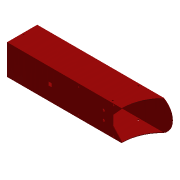
# Autodesk Inventor part: Case
Saved by Autodesk Inventor 2015 (Build 190159000, 159)
## iProperties
Created: 2015-01-07
Part Number: Case
Material: Všeobecné
Document SubType Name: Modeling
Designer: Michal
Density: 1 g/cm^3
Appearance: Červená
Author: Michal
Autodesk Inventor part; units mm, degrees
ref_plane "YZ Plane" through (0, 0, 0) normal (1, 0, 0) x (0, 1, 0)
ref_plane "XZ Plane" through (0, 0, 0) normal (0, 1, 0) x (-1, 0, 0)
ref_plane "XY Plane" through (0, 0, 0) normal (0, 0, 1) x (1, 0, 0)
sketch "Náčrt1" plane through (0, 0, 0) normal (1, 0, 0) x (0, 1, 0)
  line L0 (0, 0) -> (100, 0)
  line L1 (100, 0) -> (100, -100)
  line L2 (100, -100) -> (0, -100)
  line L3 (0, -100) -> (0, 0)
  line L4 (98, -2) -> (2, -2)
  line L5 (2, -2) -> (2, -98)
  line L6 (2, -98) -> (98, -98)
  line L7 (98, -98) -> (98, -2)
  dimension "d0" = 100
  dimension "d1" = 100
  dimension "d2" = 2
  constraints: 16 end point, 4 parallel, 2 perpendicular, 1 horizontal, 3 other
  measures "d0" distance of L1.end L2.end
  measures "d1" distance of L0.end L1.end
  measures "d2" distance between parallel lines of L0 L4
extrude "Vysunutí1" add sketch "Náčrt1" along normal blind 370
sketch "Náčrt4" plane through (0, 0, 0) normal (0, 0, 1) x (1, 0, 0)
  line L0 (0, 0) -> (0, 100) projected
  line L1 (0, 0) -> (370, 0) projected
  line L2 (370, 100) -> (370, 0) projected
  line L3 (0, 100) -> (370, 100) projected
  line L4 (0, 2) -> (370, 2) projected
  arc A0 (370, 98) -> (330.0148, 0) centre (465.2, 2) ccw
  line L5 (330, 23.5767) -> (330, -17.4459)
  line L6 (370, 2) -> (523.9799, 2)
  line L7 (330, 2) -> (370, 2)
  line L8 (0, 0) -> (370, 0) projected
  line L9 (370, 2) -> (370, 98)
  dimension "d17" = 2
  dimension "d102" = 330
  constraints: 8 end point, 5 point on line, 2 point on circle, 2 vertical, 1 centre point, 1 horizontal, 1 parallel, 1 tangent
  measures "d17" distance from line of L3 L9.end
  measures "d102" distance from line of L0 L7.start
extrude "Vysunutí4" cut sketch "Náčrt4" against normal through all contours A0 L2 L4 | L4 L2 L1 A0
sketch "Náčrt5" plane through (0, 100, 0) normal (0, 1, 0) x (1, 0, 0)
  line L0 (0, 0) -> (0, 100) projected
  line L1 (0, 0) -> (370, 0) projected
  line L2 (370, 100) -> (370, 0) projected
  line L3 (0, 100) -> (370, 100) projected
  arc A0 (370, 0) -> (370, 100) centre (343.3333, 50) ccw
  point P0 (400, 50)
  dimension "d21" = 30
  constraints: 3 point on circle, 1 centre point
  measures "d21" distance from line of point (400, 50) L2
extrude "Vysunutí5" add sketch "Náčrt5" against normal blind 2 contours L2 A0
sketch "Náčrt11" plane through (0, 0, -100) normal (0, -1, 0) x (1, 0, 0)
  line L0 (0, 100) -> (330.0148, 100) projected
  line L1 (0, 0) -> (0, 100) projected
  line L2 (0, 0) -> (330.0148, 0) projected
  line L3 (330.0148, 0) -> (330.0148, 100) projected
  line L4 (86.35, 55.65) -> (97.65, 55.65)
  line L5 (97.65, 55.65) -> (97.65, 44.35)
  line L6 (97.65, 44.35) -> (86.35, 44.35)
  line L7 (86.35, 44.35) -> (86.35, 55.65)
  point P0 (92, 55.65)
  point P1 (86.35, 50)
  dimension "d129" = 11.3
  dimension "d130" = 11.3
  dimension "d131" = 92
  dimension "d132" = 50
  constraints: 8 end point, 2 midpoint, 2 parallel, 1 horizontal, 1 perpendicular
  measures "d129" distance of L4.start L4.end
  measures "d130" distance of L4.end L5.end
  measures "d131" distance from line of L1 point (92, 55.65)
  measures "d132" distance from line of L0 point (86.35, 50)
extrude "Vysunutí11" cut sketch "Náčrt11" against normal blind 5 contours L4 L5 L6 L7
sketch "Náčrt12" plane through (0, 0, -100) normal (0, -1, 0) x (1, 0, 0)
  line L0 (0, 100) -> (330.0148, 100) projected
  line L1 (0, 0) -> (0, 100) projected
  line L2 (0, 0) -> (330.0148, 0) projected
  circle A0 centre (187, 90) radius 2.25
  circle A1 centre (187, 10) radius 2.25
  line L3 (330.0148, 0) -> (330.0148, 100) projected
  dimension "d61" = 4.5
  dimension "d62" = 4.5
  dimension "d63" = 10
  dimension "d64" = 10
  dimension "d65" = 187
  dimension "d66" = 187
  constraints: 2 centre point
  measures "d61" diameter of A0
  measures "d62" diameter of A1
  measures "d63" distance from line of L0 A0.centre
  measures "d64" distance from line of L2 A1.centre
  measures "d65" distance from line of L1 A1.centre
  measures "d66" distance from line of L1 A0.centre
extrude "Vysunutí12" cut sketch "Náčrt12" against normal blind 10 contours A0 | A1
sketch "Náčrt14" plane through (0, 0, -100) normal (0, 0, -1) x (-1, 0, 0)
  line L0 (0, 0) -> (-330.0148, 0) projected
  line L1 (0, 100) -> (0, 0) projected
  line L2 (0, 100) -> (-370, 100) projected
  line L3 (-370, 98) -> (-370, 100) projected
  circle A0 centre (-293, 7.5) radius 2.25
  circle A1 centre (-293, 92.5) radius 2.25
  arc A2 (-330.0148, 0) -> (-370, 98) centre (-465.2, 2) ccw projected
  dimension "d77" = 293
  dimension "d78" = 4.5
  dimension "d79" = 4.5
  dimension "d80" = 293
  dimension "d86" = 85
  dimension "d87" = 7.5
  constraints: 2 centre point
  measures "d77" distance from line of L1 A0.centre
  measures "d78" diameter of A0
  measures "d79" diameter of A1
  measures "d80" distance from line of L1 A1.centre
  measures "d86" distance of A0.centre A1.centre
  measures "d87" distance from line of L2 A1.centre
extrude "Vysunutí14" cut sketch "Náčrt14" against normal through all contours A0 | A1
sketch "Náčrt16" plane through (0, 0, -100) normal (0, -1, 0) x (1, 0, 0)
  circle A0 centre (187, 90) radius 2.25 projected
  circle A1 centre (187, 10) radius 2.25 projected
  line L0 (330.0148, 0) -> (330.0148, 100) projected
  line L1 (0, 100) -> (330.0148, 100) projected
  line L2 (0, 0) -> (0, 100) projected
  line L3 (0, 0) -> (330.0148, 0) projected
  line L4 (0, 2) -> (330, 2) projected
  line L5 (0, 98) -> (330, 98) projected
  line L6 (300.0148, 65) -> (300.0148, 35)
  line L7 (300.0148, 35) -> (330, 2)
  line L8 (330, 2) -> (332.6841, 2)
  line L9 (332.6841, 2) -> (332.6841, 98)
  line L10 (332.6841, 98) -> (330, 98)
  line L11 (300.0148, 65) -> (330, 98)
  circle A2 centre (303.0148, 5) radius 2.5
  circle A3 centre (303.0148, 95) radius 2.5
  point P0 (300.0148, 50)
  dimension "d103" = 30
  dimension "d104" = 50
  dimension "d105" = 30
  dimension "d106" = 5
  dimension "d107" = 5
  dimension "d108" = 5
  dimension "d109" = 5
  dimension "d110" = 27
  dimension "d111" = 27
  constraints: 12 end point, 2 centre point, 1 horizontal, 1 midpoint, 1 parallel, 1 perpendicular, 1 vertical
  measures "d103" distance of L6.start L6.end
  measures "d104" distance from line of L1 point (300.015, 50)
  measures "d105" distance between parallel lines of L0 L6
  measures "d106" diameter of A2
  measures "d107" diameter of A3
  measures "d108" distance from line of L3 A2.centre
  measures "d109" distance from line of L1 A3.centre
  measures "d110" distance from line of L0 A2.centre
  measures "d111" distance from line of L0 A3.centre
extrude "Vysunutí17" cut sketch "Náčrt16" against normal up to surface (2 mm away) contours L8 L7 L6 L11 L10 L0 | L0 L10 L9 L8 | A2 | A3
sketch "Náčrt17" plane through (0, 0, 0) normal (-1, 0, 0) x (0, 0, 1)
  line L0 (-98, 98) -> (-2, 98) projected
  line L1 (-2, 98) -> (-2, 2) projected
  line L2 (-2, 2) -> (-98, 2) projected
  line L3 (-98, 2) -> (-98, 98) projected
  line L4 (0, 0) -> (0, 100) projected
  line L5 (0, 100) -> (-100, 100) projected
  line L6 (-100, 100) -> (-100, 0) projected
  line L7 (-100, 0) -> (0, 0) projected
extrude "Vysunutí18" add sketch "Náčrt17" along normal blind 50
sketch "Náčrt18" plane through (-50, 100, 0) normal (0, 0, 1) x (1, 0, 0)
  arc A0 (420, -2) -> (380.0148, -100) centre (515.2, -98) ccw projected
  line L0 (420, 0) -> (420, -2) projected
  line L1 (420, 0) -> (0, 0) projected
  line L2 (0, -100) -> (0, 0) projected
  line L3 (0, -100) -> (380.0148, -100) projected
  circle A1 centre (5, -50) radius 1.75
  point P0 (50, -100)
  dimension "d116" = 3.5
  dimension "d117" = 50
  dimension "d118" = 5
  constraints: 1 centre point
  measures "d116" diameter of A1
  measures "d117" distance from line of L3 A1.centre
  measures "d118" distance from line of L2 A1.centre
extrude "Vysunutí19" cut sketch "Náčrt18" against normal through all contours A1
sketch "Náčrt19" plane through (300.0148, 0, -65) normal (0, -1, 0) x (1, 0, 0)
  line L0 (29.9852, 63) -> (30, 63) projected
  line L1 (30, 63) -> (30, 65) projected
  line L2 (-350.0148, 65) -> (30, 65) projected
  line L3 (-350.0148, -35) -> (-350.0148, 65) projected
  line L4 (30, -35) -> (-350.0148, -35) projected
  line L5 (30, -35) -> (30, -33) projected
  line L6 (30, -33) -> (29.9852, -33) projected
  line L7 (29.9852, -33) -> (0, 0) projected
  line L8 (0, 0) -> (0, 30) projected
  line L9 (0, 30) -> (29.9852, 63) projected
  circle A0 centre (3, 60) radius 2.5 projected
  circle A1 centre (3, -30) radius 2.5 projected
  circle A2 centre (-113.0148, 55) radius 2.25 projected
  circle A3 centre (-113.0148, -25) radius 2.25 projected
  circle A4 centre (-30, 29.5) radius 4
  circle A5 centre (-30, 0.5) radius 4
  point P0 (-300.0148, 65)
  dimension "d121" = 8
  dimension "d122" = 8
  dimension "d123" = 29
  dimension "d124" = 35.5
  dimension "d125" = 30
  dimension "d126" = 30
  constraints: 2 centre point
  measures "d121" diameter of A4
  measures "d122" diameter of A5
  measures "d123" distance of A5.centre A4.centre
  measures "d124" distance from line of L2 A4.centre
  measures "d125" distance from line of A5.centre L8
  measures "d126" distance from line of L8 A4.centre
extrude "Vysunutí20" cut sketch "Náčrt19" against normal blind 10 contours A4 | A5
